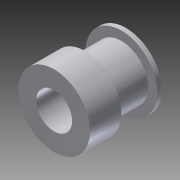
# Autodesk Inventor part: Timping Pully
Saved by Autodesk Inventor 2014 (Build 180170000, 170)
## iProperties
Created: 2013-12-16
Part Number: Timping Pully
Material: Aluminum
Document SubType Name: Modeling
Designer: Bram
Density: 2.71 g/cm^3
Appearance: Satin
Author: Bram
Autodesk Inventor part; units mm, degrees
ref_plane "YZ Plane" through (0, 0, 0) normal (1, 0, 0) x (0, 1, 0)
ref_plane "XZ Plane" through (0, 0, 0) normal (0, 1, 0) x (-1, 0, 0)
ref_plane "XY Plane" through (0, 0, 0) normal (0, 0, 1) x (1, 0, 0)
sketch "Sketch1" plane through (0, 0, 0) normal (0, 1, 0) x (-1, 0, 0)
  circle A0 centre (0, 0) radius 8
  circle A1 centre (0, 0) radius 4
  dimension "d0" = 16
  dimension "d1" = 8
  constraints: 2 centre point, 2 coincident
  measures "d0" diameter of A0
  measures "d1" diameter of A1
extrude "Extrusion1" add sketch "Sketch1" along normal blind 15
sketch "Sketch2" plane through (0, 15, 0) normal (0, 1, 0) x (1, 0, 0)
  circle A0 centre (0, 0) radius 8 projected
  circle A1 centre (0, 0) radius 6
  dimension "d4" = 12
  constraints: 1 centre point, 1 coincident
  measures "d4" diameter of A1
extrude "Extrusion2" cut sketch "Sketch2" against normal blind 8
sketch "Sketch3" plane through (0, 15, 0) normal (0, 1, 0) x (1, 0, 0)
  circle A0 centre (0, 0) radius 4 projected
  circle A1 centre (0, 0) radius 8
  dimension "d7" = 16
  constraints: 1 centre point, 1 coincident
  measures "d7" diameter of A1
extrude "Extrusion3" add sketch "Sketch3" along normal blind 1
body "Solid1"
